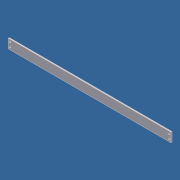
# Autodesk Inventor part: BackStrap1
Saved by Autodesk Inventor 2012 SP1 (Build 160190100, 190)
## iProperties
Created: 2010-12-15
Part Number: BackStrap1
Document SubType Name: Modeling
Designer: berny
Density: 2.71 g/cm^3
Material: Aluminum-6061
Mass: 98.0283 g
Surface Area: 259.825 cm^2
Volume: 36.1728 cm^3
Author: berny
Autodesk Inventor part; units mm, degrees
ref_plane "YZ Plane" through (0, 0, 0) normal (1, 0, 0) x (0, 1, 0)
ref_plane "XZ Plane" through (0, 0, 0) normal (0, 1, 0) x (-1, 0, 0)
ref_plane "XY Plane" through (0, 0, 0) normal (0, 0, 1) x (1, 0, 0)
sketch "Sketch1" plane through (0, 0, 0) normal (0, 0, 1) x (1, 0, 0)
  line L0 (0, 0) -> (450.85, 0)
  line L1 (450.85, 0) -> (450.85, 25.4)
  line L2 (450.85, 25.4) -> (0, 25.4)
  line L3 (0, 25.4) -> (0, 0)
  dimension "d0" = 25.4
  dimension "d1" = 450.85
  constraints: 8 end point, 2 parallel, 1 horizontal, 1 perpendicular
  measures "d0" distance between parallel lines of L0 L2
  measures "d1" distance between parallel lines of L1 L3
extrude "Extrusion1" add sketch "Sketch1" along normal blind 3.175
sketch "Sketch2" plane through (0, 0, 3.175) normal (0, 0, 1) x (1, 0, 0)
  line L0 (0, 0) -> (0, 25.4) projected
  line L1 (450.85, 0) -> (0, 0) projected
  line L2 (450.85, 25.4) -> (450.85, 0) projected
  line L3 (0, 25.4) -> (450.85, 25.4) projected
  point P0 (4.7625, 19.05)
  point P1 (4.7625, 6.35)
  point P2 (446.0875, 6.35)
  point P3 (446.0875, 19.05)
  dimension "d4" = 6.35
  dimension "d5" = 6.35
  dimension "d6" = 4.7625
  dimension "d7" = 4.7625
  constraints: 2 horizontal alignment, 2 vertical alignment
  measures "d4" distance from line of L1 point (4.763, 6.35)
  measures "d5" distance from line of L3 point (4.763, 19.05)
  measures "d6" distance from line of L0 point (4.763, 6.35)
  measures "d7" distance from line of point (446.087, 6.35) L2
hole "Hole1" at (4.7625, 19.05, 3.175) at (4.7625, 6.35, 3.175) at (446.0875, 6.35, 3.175) at (446.0875, 19.05, 3.175) direction (0, 0, -1) diameter 4.318 end through all clearance for "Socket Head Cap Screw" size "#8" standard "Ansi Unified Screw Threads"
body "Solid1"
